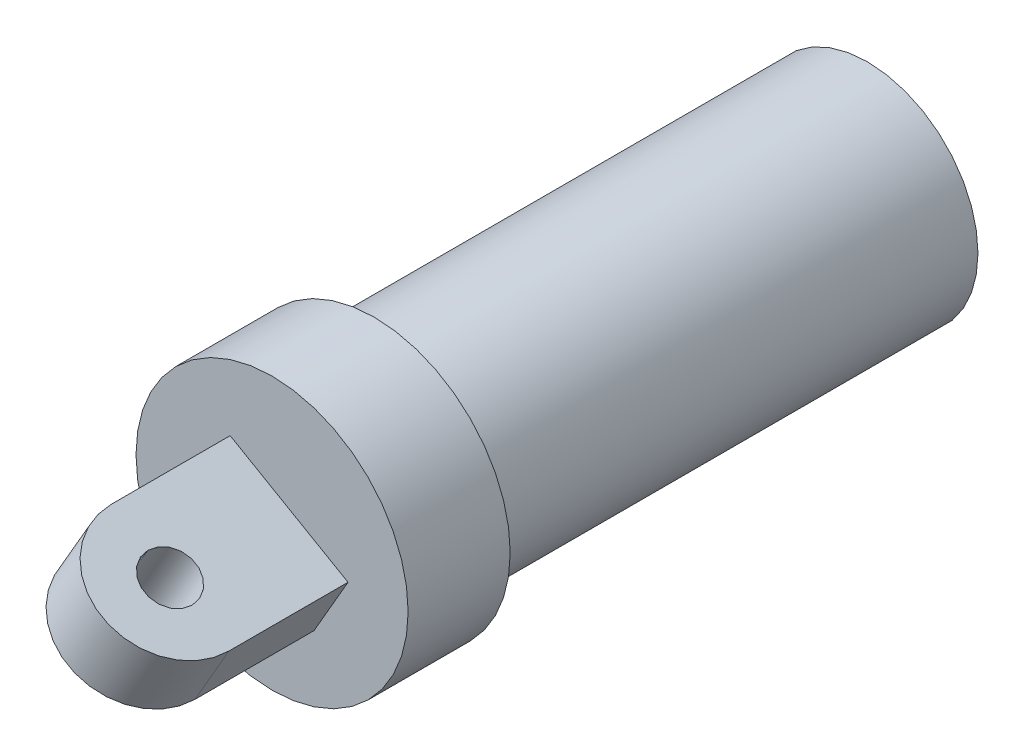
# Autodesk Inventor part: ダンパー上パーツ
Saved by Autodesk Inventor 2020.2 (Build 242310000, 310)
## iProperties
Created: 2018-03-29
Part Number: ダンパー上パーツ
Material: 一般
Document SubType Name: Modeling
Designer: Takumi
Density: 1 g/cm^3
Appearance: ポリカーボネート - スモーク
Mass: 5.14688 g
Surface Area: 24.2151 cm^2
Volume: 5.14688 cm^3
Author: Takumi
Autodesk Inventor part; units mm, degrees
ref_plane "YZ Plane" through (0, 0, 0) normal (1, 0, 0) x (0, 1, 0)
ref_plane "XZ Plane" through (0, 0, 0) normal (0, 1, 0) x (-1, 0, 0)
ref_plane "XY Plane" through (0, 0, 0) normal (0, 0, 1) x (1, 0, 0)
sketch "スケッチ1" plane through (0, 0, 0) normal (0, 0, 1) x (1, 0, 0)
  line L0 (0, 7.5056) -> (6.5, 3.7528)
  line L1 (6.5, 3.7528) -> (6.5, -3.7528)
  line L2 (6.5, -3.7528) -> (0, -7.5056)
  line L3 (0, -7.5056) -> (-6.5, -3.7528)
  line L4 (-6.5, -3.7528) -> (-6.5, 3.7528)
  line L5 (-6.5, 3.7528) -> (0, 7.5056)
  circle A0 centre (0, 0) radius 6.5
  dimension "d0" = 13
  dimension "d1" = 13
  constraints: 12 end point, 2 coincident, 1 centre point, 13 other
  measures "d0" distance between parallel lines of L3 L0
  measures "d1" diameter of A0
extrude "押し出し1" add sketch "スケッチ1" along normal blind 6
extrude "押し出し2" add sketch "スケッチ1" against normal blind 29 contours A0
ref_plane "作業平面1" through (-3.25, 1.8764, 6) normal (0.5, 0.8660254, 0) x (0.8660254, -0.5, 0)
sketch "スケッチ2" plane through (-3.25, 1.8764, 6) normal (0.5, 0.8660254, 0) x (0.8660254, -0.5, 0)
  line L0 (0, 6) -> (3.7528, 6) projected
  line L1 (0, 6) -> (0, 0) projected
  line L2 (7.5056, 0) -> (0, 0) projected
  line L3 (7.5056, 6) -> (7.5056, 0) projected
  line L4 (3.7528, 6) -> (3.7528, -7)
  line L5 (3.7528, -7) -> (3.7528, 0) construction
  line L6 (7.7528, -7) -> (7.7528, 0)
  line L7 (-0.2472, 0) -> (-0.2472, -7)
  arc A0 (-0.2472, -7) -> (7.7528, -7) centre (3.7528, -7) ccw
  arc A1 (7.7528, 0) -> (-0.2472, 0) centre (3.7528, 0) ccw
  line L8 (3.7528, 6) -> (7.5056, 6) projected
  point P0 (3.7528, -3.5)
  dimension "d7" = 7
  dimension "d8" = 8
  constraints: 10 end point, 4 point on circle, 4 tangent, 2 centre point, 2 midpoint, 1 parallel, 1 point on line, 1 vertical
  measures "d7" distance from line of L4.end L2
  measures "d8" diameter of A1
extrude "押し出し3" add sketch "スケッチ2" along normal mid plane 4 contours A1 L4 L2 L1 | L1 L2 L3 A1 L6 A0 L7 | A1 L3 L2 L4
hole "穴1" at (0, 0, 13) direction (0.5, 0.8660254, 0) diameter 3 end through all
hole "穴2" at (0, 0, 13) direction (-0.5, -0.8660254, 0) diameter 3 end through all
hole "穴3" at (0, 0, 0) direction (0, 0, -1) diameter 3 end through all
sketch "スケッチ3" plane through (0, 0, 6) normal (0, 0, 1) x (1, 0, 0)
  circle A0 centre (0, 0) radius 1.5 projected
  circle A1 centre (0, 0) radius 8
  dimension "d32" = 16
  constraints: 1 centre point, 1 coincident
  measures "d32" diameter of A1
extrude "押し出し4" add sketch "スケッチ3" against normal blind 6
